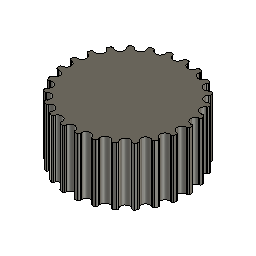
HTD-5M Generator (Autodesk Fusion 360 design; units mm, degrees)
Autodesk Fusion 360 part; units mm, degrees
note: some values were not read from the file. Set by a fixed rule: which sketch regions a step uses.
sketch "Teeth" plane through (0, 0, 0) normal (0, 0, 1) x (1, 0, 0)
  circle A0 centre (0, 0) radius 19.8944
  arc A1 (0.3922, 19.0203) -> (0, 19.0244) centre (0, 0) ccw
  arc A2 (0.8131, 18.6038) -> (0.3922, 19.0203) centre (0.3833, 18.5904) ccw
  line L0 (0.8131, 18.6038) -> (0.8237, 18.2627)
  arc A3 (0.8237, 18.2627) -> (2.1262, 16.8306) centre (2.3129, 18.3089) ccw
  line L1 (0, 0) -> (0, 19.0244) construction
  line L2 (0, 0) -> (2.3129, 18.3089) construction
  line L3 (0, 19.0244) -> (0, 19.8944)
  arc A4 (2.4934, 19.7375) -> (0, 19.8944) centre (0, 0) ccw
  arc A5 (2.1262, 16.8306) -> (3.744, 17.8937) centre (2.3129, 18.3089) ccw
  line L4 (3.839, 18.2215) -> (3.744, 17.8937)
  arc A6 (4.3503, 18.5203) -> (3.839, 18.2215) centre (4.252, 18.1017) ccw
  arc A7 (4.7312, 18.4267) -> (4.3503, 18.5203) centre (0, 0) ccw
  line L5 (4.7312, 18.4267) -> (4.9475, 19.2694)
  arc A8 (4.9475, 19.2694) -> (2.4934, 19.7375) centre (0, 0) ccw
  line L6 (0.8131, 18.6038) -> (2.3261, 18.4126) construction
  line L7 (2.3261, 18.4126) -> (2.3129, 18.3089) construction
  dimension "d50" = 39.7888
  dimension "d57" = 0.43
  dimension "d58" = 1.49
  dimension "d59" = 7.2
  dimension "d62" = 2.93
  dimension "d65" = 0.87
  dimension "d67" = 1.525
  constraint tangent A1 A2
  constraint coincident A0.centre A1.centre
  constraint vertical A0.centre A1.end
  constraint coincident A0 L3.end
  constraint parallel L1 L3
  constraint coincident A0 A4.start
  constraint collinear A3.centre A0.centre A4.start
  constraint coincident A3.centre L2.end
  constraint coincident L2 A3.end
  constraint symmetric L0.end L2 A5.end
  constraint symmetric A2.start L2 L4.start
  constraint symmetric A1.start L2 A6.start
  constraint symmetric A1 L2 A7
  constraint symmetric A2 L2 A6
  constraint symmetric A3 L2 A5
  constraint symmetric L2 A1.end A7.start
  constraint symmetric L2 L3.end L5.end
  constraint symmetric L2 A4.start A8.end
  constraint symmetric L2 A4 A8
  constraint symmetric L2 A3.end A5.start
  constraint tangent L0 A3
  constraint tangent A2 L0
  constraint perpendicular L2 L6
  constraint parallel L2 L7
  measures "d50" diameter of A0
  measures "d57" radius of A2
  measures "d58" radius of A3
  measures "d59" angle of L1 L2
  measures "d62" distance of A4.start A3.end
  measures "d65" distance of A1.end L3.end
  measures "d67" distance of A2.start L6.end
extrude "Extrude1" add sketch "Teeth" along normal mid plane 18.5
extrude "Extrude3" cut sketch "Teeth" along normal through all and the other way through all contours A0 A1 A2 L0 A3 L3 A4 A5 L4 A6 A7 L5 A8
pattern_circular "C-Pattern1" count 25 over 360 about axis through (0, 0, 0) along (0, 0, 1) of "Extrude3"
equation "p = 5 mm"
equation "Dr = 0.2 in" comment "0.13 for #25, 0.2 for #35"
equation "Ds = 1.0005 * Dr + 0.003 in"
equation "n = 25" comment "Number of Teeth"
equation "PD = n * p / 3.14159"
equation "A_angle = 35 deg + ( 60 / n ) * 1 deg"
equation "B_angle = 18 deg - ( 56 / n ) * 1 deg"
equation "ac = 0.8 * Dr"
equation "ab = 1.4 * Dr"
equation "OD = PD + 0.55 * p"
equation "d25 = width"
equation "d50 = PD"
equation "d52 = n"
equation "d59 = ( 180 / n ) * 1 deg"
equation "width = 18.5 mm"
equation "d67 = 3.05 mm / 2"
